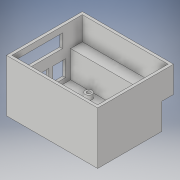
# Autodesk Inventor part: MainPCB_RPI_Case
Saved by Autodesk Inventor 2019.4 (Build 234330000, 330)
## iProperties
Created: 2020-03-12
Part Number: MainPCB_RPI_Case
Material: Generic
Document SubType Name: Modeling
Designer: Jorian Bruslind
Density: 1 g/cm^3
Appearance: Default
Author: Jorian Bruslind
Autodesk Inventor part; units mm, degrees
ref_plane "YZ Plane" through (0, 0, 0) normal (1, 0, 0) x (0, 1, 0)
ref_plane "XZ Plane" through (0, 0, 0) normal (0, 1, 0) x (-1, 0, 0)
ref_plane "XY Plane" through (0, 0, 0) normal (0, 0, 1) x (1, 0, 0)
sketch "Sketch1" plane through (0, 0, 0) normal (0, 1, 0) x (-1, 0, 0)
  line L0 (0, 0) -> (95, 0)
  line L1 (95, 0) -> (95, -65)
  line L2 (95, -65) -> (0, -65)
  line L3 (0, -65) -> (0, 0)
  line L4 (98, -68) -> (98, 3)
  line L5 (98, 3) -> (-3, 3)
  line L6 (-3, 3) -> (-3, -68)
  line L7 (-3, -68) -> (98, -68)
  dimension "d0" = 95
  dimension "d1" = 65
  dimension "d2" = 3
  constraints: 16 end point, 4 parallel, 2 perpendicular, 1 horizontal, 3 other
  measures "d0" distance of L1.end L2.end
  measures "d1" distance of L0.end L1.end
  measures "d2" distance between parallel lines of L1 L4
extrude "Extrusion1" add sketch "Sketch1" along normal blind 32 contours L0 L1 L2 L3 | L7 L6 L5 L4
sketch "Sketch2" plane through (0, 32, 0) normal (0, 1, 0) x (1, 0, 0)
  line L0 (0, 0) -> (-95, 0)
  line L1 (-95, 0) -> (-95, 65)
  line L2 (-95, 65) -> (0, 65)
  line L3 (0, 65) -> (0, 0)
  dimension "d5" = 95
  dimension "d6" = 65
  constraints: 8 end point, 2 parallel, 1 horizontal, 1 perpendicular
  measures "d5" distance of L1.end L2.end
  measures "d6" distance of L0.end L1.end
extrude "Extrusion2" cut sketch "Sketch2" against normal blind 30
sketch "Sketch3" plane through (0, 2, 0) normal (0, 1, 0) x (1, 0, 0)
  line L0 (0, 65) -> (0, 0) projected
  line L1 (0, 0) -> (0, 9)
  line L2 (0, 9) -> (-10, 9)
  circle A0 centre (-10, 9) radius 2
  circle A1 centre (-10, 9) radius 4
  circle A2 centre (-10, 58) radius 4
  circle A3 centre (-10, 58) radius 2
  circle A4 centre (-68, 9) radius 4
  circle A5 centre (-68, 9) radius 2
  circle A6 centre (-68, 58) radius 4
  circle A7 centre (-68, 58) radius 2
  dimension "d9" = 9
  dimension "d10" = 10
  dimension "d11" = 4
  dimension "d12" = 8
  dimension "d15" = 49
  dimension "d18" = 58
  constraints: 8 centre point, 5 coincident, 4 end point, 1 horizontal, 1 perpendicular, 1 point on line, 1 vertical, 12 other
  measures "d9" distance of L0.end L1.end
  measures "d10" distance of L1.end L2.end
  measures "d11" diameter of A0
  measures "d12" diameter of A1
  measures "d15" distance of A1.centre A2.centre
  measures "d18" distance of A1.centre A4.centre
extrude "Extrusion3" add sketch "Sketch3" along normal blind 5
sketch "Sketch4" plane through (0, 32, 0) normal (0, 1, 0) x (1, 0, 0)
  line L0 (3, 68) -> (-98, 68) projected
  line L1 (3, 68) -> (-98, 68)
  line L2 (-98, 68) -> (-98, 81)
  line L3 (-98, 81) -> (3, 81)
  line L4 (3, 81) -> (3, 68)
  point P0 (0, 0)
  dimension "d23" = 13
  dimension "d62" = 101
  constraints: 8 end point, 2 parallel, 1 horizontal, 1 perpendicular
  measures "d23" distance of L1.end L2.end
  measures "d62" distance of L2.end L3.end
extrude "Extrusion4" add sketch "Sketch4" against normal blind 3
sketch "Sketch5" plane through (0, 32, 0) normal (0, 1, 0) x (1, 0, 0)
  line L0 (-98, 81) -> (3, 81) projected
  line L1 (3, 81) -> (-97, 81)
  line L2 (-97, 81) -> (-97, 78)
  line L3 (-97, 78) -> (3, 78)
  line L4 (3, 78) -> (3, 81)
  line L5 (3, 81) -> (0, 81)
  line L6 (0, 81) -> (0, -3)
  line L7 (0, -3) -> (3, -3)
  line L8 (3, -3) -> (3, 81)
  line L9 (-98, 68) -> (-98, 81) projected
  line L10 (-98, 81) -> (-95, 81)
  line L11 (-95, 81) -> (-95, -3)
  line L12 (-95, -3) -> (-98, -3)
  line L13 (-98, -3) -> (-98, 81)
  line L14 (-98, -3) -> (2, -3)
  line L15 (2, -3) -> (2, 0)
  line L16 (2, 0) -> (-98, 0)
  line L17 (-98, 0) -> (-98, -3)
  point P0 (0, 0)
  dimension "d26" = 100
  dimension "d27" = 3
  dimension "d28" = 3
  dimension "d29" = 84
  dimension "d30" = 3
  dimension "d31" = 84
  dimension "d32" = 100
  dimension "d33" = 3
  constraints: 32 end point, 8 parallel, 4 horizontal, 4 perpendicular, 1 other
  measures "d26" distance of L3.end L2.end
  measures "d27" distance of L2.end L1.end
  measures "d28" distance of L7.end L6.end
  measures "d29" distance of L6.end L5.end
  measures "d30" distance of L11.end L12.end
  measures "d31" distance of L10.end L11.end
  measures "d32" distance of L16.end L15.end
  measures "d33" distance of L15.end L14.end
extrude "Extrusion5" add sketch "Sketch5" along normal blind 26 contours L0 L2 L3 L11 L16 L13 L9 | L0 L11 L3 L2 | L0 L6 L3 L11 | L16 L11 L12 L13 | L0 L4 L3 L6 | L16 L6 L14 L11 | L3 L8 L7 L15 L16 L6 | L16 L15 L7 L6
sketch "Sketch6" plane through (-98, 0, -68) normal (-1, 0, 0) x (0, 0, 1)
  line L0 (71, 0) -> (71, 32) projected
  line L1 (71, 58) -> (61.858, 58)
  line L2 (71, 58) -> (-13, 58) projected
  line L3 (61.858, 58) -> (61.858, 51.5)
  line L4 (61.858, 51.5) -> (11.858, 51.5)
  line L5 (11.858, 51.5) -> (11.858, 36.5)
  line L6 (11.858, 36.5) -> (61.858, 36.5)
  line L7 (61.858, 36.5) -> (61.858, 51.5)
  line L8 (3, 32) -> (3, 2) projected
  line L9 (3, 2) -> (3, 7)
  line L10 (68, 2) -> (3, 2) projected
  line L11 (3, 2) -> (8, 2) construction
  line L12 (3, 7) -> (8.54, 7)
  line L13 (8.54, 7) -> (22.54, 7)
  line L14 (22.54, 7) -> (22.54, 25)
  line L15 (22.54, 25) -> (8.54, 25)
  line L16 (8.54, 25) -> (8.54, 7)
  line L17 (22.54, 7) -> (27.04, 7)
  line L18 (27.04, 7) -> (41.04, 7)
  line L19 (41.04, 7) -> (41.04, 25)
  line L20 (41.04, 25) -> (27.04, 25)
  line L21 (27.04, 25) -> (27.04, 7)
  point P0 (68, 0)
  dimension "d36" = 9.142
  dimension "d37" = 6.5
  dimension "d38" = 50
  dimension "d39" = 15
  dimension "d40" = 5
  dimension "d41" = 90
  dimension "d42" = 5.54
  dimension "d43" = 14
  dimension "d44" = 18
  dimension "d45" = 4.5
  dimension "d46" = 14
  dimension "d47" = 18
  constraints: 36 end point, 7 perpendicular, 6 parallel, 5 horizontal, 1 point on line
  measures "d36" distance of L1.start L1.end
  measures "d37" distance of L1.end L3.end
  measures "d38" distance of L6.end L5.end
  measures "d39" distance of L5.end L4.end
  measures "d40" distance of L8.end L9.end
  measures "d41" angle of L11 L9
  measures "d42" distance of L9.end L12.end
  measures "d43" distance of L15.end L14.end
  measures "d44" distance of L14.end L13.end
  measures "d45" distance of L13.end L17.end
  measures "d46" distance of L20.end L19.end
  measures "d47" distance of L19.end L18.end
extrude "Extrusion6" cut sketch "Sketch6" against normal blind 3
sketch "Sketch7" plane through (3, 0, -68) normal (0, 0, -1) x (-1, 0, 0)
  line L0 (3, 2) -> (3, 32) projected
  line L1 (3, 2) -> (4, 2)
  line L2 (4, 2) -> (4, 7)
  line L3 (4, 7) -> (31.75, 7)
  line L4 (31.75, 7) -> (39.75, 7)
  line L5 (39.75, 7) -> (39.75, 11)
  line L6 (39.75, 11) -> (31.75, 11)
  line L7 (31.75, 11) -> (31.75, 7)
  point P0 (3, 0)
  point P1 (3, 58)
  dimension "d50" = 1
  dimension "d51" = 5
  dimension "d52" = 27.75
  dimension "d53" = 8
  dimension "d54" = 4
  constraints: 14 end point, 3 horizontal, 2 parallel, 2 perpendicular
  measures "d50" distance of L0.start L1.end
  measures "d51" distance of L1.end L2.end
  measures "d52" distance of L2.end L3.end
  measures "d53" distance of L6.end L5.end
  measures "d54" distance of L5.end L4.end
extrude "Extrusion7" cut sketch "Sketch7" against normal blind 3
body "Solid1"
